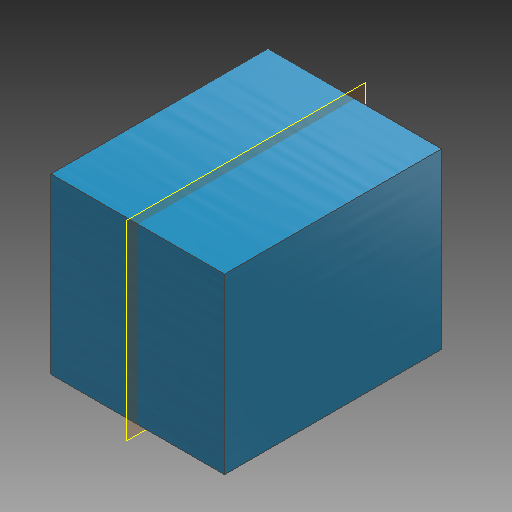
# Autodesk Inventor part: aandrijfMotor
Saved by Autodesk Inventor 2017 (Build 210142000, 142)
## iProperties
Created: 2017-02-17
Part Number: aandrijfMotor
Material: Generic
Document SubType Name: Modeling
Designer: Koen
Density: 1 g/cm^3
Appearance: Default
Author: Koen
Autodesk Inventor part; units mm, degrees
ref_plane "YZ Plane" through (0, 0, 0) normal (1, 0, 0) x (0, 1, 0)
ref_plane "XZ Plane" through (0, 0, 0) normal (0, 1, 0) x (-1, 0, 0)
ref_plane "XY Plane" through (0, 0, 0) normal (0, 0, 1) x (1, 0, 0)
sketch "Sketch1" plane through (0, 0, 0) normal (0, 0, 1) x (1, 0, 0)
  line L0 (700, -200) -> (180, -200) projected
  line L1 (180, -200) -> (-160, -200) projected
  line L2 (-160, -200) -> (-160, 200) projected
  line L3 (180, -200) -> (180, 200) projected
  line L4 (700, -200) -> (1018.8395, -200) projected
  line L5 (1018.8395, -200) -> (1018.8395, 200) projected
  line L6 (1018.8395, 200) -> (700, 200) projected
  line L7 (180, 200) -> (700, 200) projected
  line L8 (-160, 200) -> (180, 200) projected
  line L9 (740, 160) -> (740, 200) projected
  line L10 (740, 160) -> (740, -160) projected
  line L11 (740, -200) -> (740, -160) projected
  line L12 (700, 160) -> (700, -160) projected
  line L13 (700, -160) -> (700, -200) projected
  line L14 (700, 200) -> (700, 160) projected
  line L15 (140, 160) -> (140, 200) projected
  line L16 (140, -200) -> (140, -160) projected
  line L17 (140, 160) -> (140, -160) projected
  line L18 (700, -160) -> (180, -160) projected
  line L19 (180, 160) -> (700, 160) projected
  line L20 (180, -200) -> (340, -200)
  line L21 (340, -200) -> (340, 0)
  line L22 (340, 0) -> (180, 0)
  line L23 (180, 0) -> (180, -200)
  point P0 (0, 0)
  point P1 (260, 0)
  point P2 (140, 0)
  dimension "d0" = 160
  constraints: 8 end point, 2 midpoint, 2 parallel, 1 horizontal, 1 horizontal alignment, 1 perpendicular
  measures "d0" distance of L22.end L21.end
extrude "Extrusion1" add sketch "Sketch1" along normal blind 160 contours L0 L3 L18 L21 | L18 L3 L22 L21
ref_plane "Work Plane1" through (260, -200, 0) normal (1, 0, 0) x (0, 0, -1)
sketch "Sketch2" plane through (260, -200, 0) normal (1, 0, 0) x (0, 0, -1)
  line L0 (0, 200) -> (0, 0) projected
  line L1 (0, 0) -> (-160, 0) projected
  line L2 (-160, 200) -> (-160, 0) projected
  line L3 (0, 200) -> (-160, 200) projected
  line L4 (0, 0) -> (-160, 0) projected
  line L5 (-80, 0) -> (-80, 200)
  line L6 (0, 200) -> (-160, 200) projected
  line L7 (-74, 200) -> (-74, 220)
  line L8 (-74, 220) -> (-50, 220)
  line L9 (-50, 220) -> (-50, 228)
  line L10 (-50, 228) -> (-80, 228)
  line L11 (-80, 228) -> (-80, 200)
  line L12 (-80, 200) -> (-80, 294.9893)
  dimension "d6" = 8
  dimension "d7" = 12
  dimension "d8" = 20
  dimension "d9" = 30
  dimension "d10" = 94.9893
  constraints: 14 end point, 4 perpendicular, 2 midpoint, 2 point on line, 1 collinear
  measures "d6" distance of L8.end L9.end
  measures "d7" diameter of L7 L5
  measures "d8" distance between parallel lines of L3 L8
  measures "d9" distance between parallel lines of L11 L9
  measures "d10" distance of L5.end L12.end
revolve "Revolution1" add sketch "Sketch2" angle 360 about axis through (260, 0, 80) along (0, 1, 0) contours L3 L11 L10 L9 L8 L7
body "Solid1"
